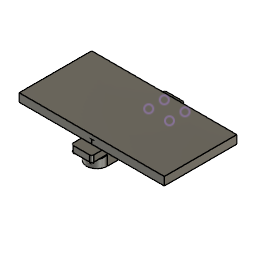
TASK-2 (Autodesk Fusion 360 design; units mm, degrees)
part number: 2026-05-20-12-53-01-030
Autodesk Fusion 360 part; units mm, degrees
sketch "rectangle" plane through (0, 0, 0) normal (0, 0, 1) x (1, 0, 0)
  line L0 (70, 35) -> (-70, 35)
  line L1 (-70, 35) -> (-70, -35)
  line L2 (-70, -35) -> (70, -35)
  line L3 (70, -35) -> (70, 35)
  line L4 (70, 35) -> (-70, -35) construction
  line L5 (-70, 35) -> (70, -35) construction
  dimension "d1" = 70
  dimension "d2" = 140
  constraint horizontal L0
  constraint perpendicular L0 L1
  constraint parallel L0 L2
  constraint parallel L1 L3
  constraint coincident L4 origin
  constraint coincident L5 origin
  measures "d1" distance of L0.end L1.end
  measures "d2" distance of L0.start L0.end
extrude "Extrude1" add sketch "rectangle" along normal blind 8
sketch "Sketch2" plane through (0, 0, 0) normal (0, 0, -1) x (1, 0, 0)
  line L0 (70, -35) -> (70, 35)
  line L1 (70, 35) -> (-70, 35)
  line L2 (-70, 35) -> (-70, -35)
  line L3 (-70, -35) -> (70, -35)
  line L4 (10, -45) -> (-10, -45)
  line L5 (-10, -45) -> (-10, 45)
  line L6 (-10, 45) -> (10, 45)
  line L7 (10, 45) -> (10, -45)
  line L8 (-6, 39) -> (-6, 21.0153)
  arc A0 (-6, 21.0153) -> (6, 21.0153) centre (0, 21.0153) ccw
  line L9 (6, 21.0153) -> (6, 39)
  arc A1 (6, 39) -> (-6, 39) centre (0, 39) ccw
  line L10 (0, 45) -> (0, 15.0153) construction
  dimension "d5" = 90
  dimension "d8" = 12
  constraint horizontal L4
  constraint perpendicular L4 L5
  constraint parallel L4 L6
  constraint parallel L5 L7
  constraint tangent L8 A0
  constraint tangent A0 L9
  constraint parallel L8 L9
  constraint tangent L9 A1
  constraint tangent L8 A1
  constraint coincident A1 L10.start
  constraint coincident A0 L10.end
  constraint coincident A0.centre L10
  constraint coincident A1.centre L10
  constraint perpendicular L3 L10
  constraint midpoint L6 L10.start
  measures "d5" distance of L4.end L5.end
  measures "d8" diameter of A0
extrude "Extrude2" add sketch "Sketch2" along normal blind 8 contours L3 L4 L5 L7 | L1 L3 L5 L7 L8 A0 L9 | L1 L6 L7 L9 A1 | L1 L8 A0 L9 | L1 L8 L9 A1 | L1 L5 L6 L8 A1
sketch "Sketch3" plane through (0, 0, -8) normal (0, 0, -1) x (1, 0, 0)
  line L0 (10, 45) -> (-10, 45)
  line L1 (-10, 45) -> (-10, -45)
  line L2 (-10, -45) -> (10, -45)
  line L3 (10, -45) -> (10, 45)
  line L4 (10, -30) -> (10, 30)
  arc A0 (10, 30) -> (-10, 30) centre (0, 30) ccw
  line L5 (-10, 30) -> (-10, -30)
  arc A1 (-10, -30) -> (10, -30) centre (0, -30) ccw
  line L6 (0, -30) -> (0, 30) construction
  constraint tangent L4 A0
  constraint tangent A0 L5
  constraint parallel L4 L5
  constraint tangent L5 A1
  constraint tangent L4 A1
  constraint perpendicular L0 L6
  constraint midpoint L6 origin
extrude "Extrude3" add sketch "Sketch3" along normal blind 8 contours L1 L3 L4 A0 L5 A1
sketch "Sketch4" plane through (0, 0, -8) normal (0, 0, -1) x (1, 0, 0)
  arc A0 (-10, -30) -> (10, -30) centre (0, -30) ccw
  line L0 (-10, -45) -> (10, -45)
hole "Hole1" at (0, -30, -16) direction (0, 0, 1) diameter 10 depth 20 tip angle 118
hole "Hole2" at (0, 30, -16) direction (0, 0, 1) diameter 10 depth 20 tip angle 118
hole "Hole3" at (0, 0, -16) direction (0, 0, 1) diameter 10 depth 20 tip angle 118
fillet "Fillet1" radius 2 3 edges at (-10, -37.5, -8) (-10, -45, -4) (0, -45, -8)
fillet "Fillet2" radius 2 3 edges at (10, -45, -3) (10, -44.4142, -7.4142) (10, -36.5, -8)
fillet "Fillet3" radius 2 2 edges at (-10, 37.5, -8) (-10, 45, -4)
fillet "Fillet4" radius 2 2 edges at (10, 37.5, -8) (10, 45, -4)
